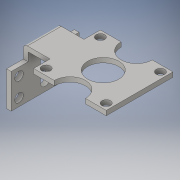
# Autodesk Inventor part: msheehan_motor_mount
Saved by Autodesk Inventor 2016 (Build 200138000, 138)
## iProperties
Created: 2017-08-31
Part Number: msheehan_motor_mount
Material: Generic
Document SubType Name: Modeling
Designer: Student
Density: 1 g/cm^3
Appearance: Default
Author: Student
Autodesk Inventor part; units mm, degrees
ref_plane "YZ Plane" through (0, 0, 0) normal (1, 0, 0) x (0, 1, 0)
ref_plane "XZ Plane" through (0, 0, 0) normal (0, 1, 0) x (-1, 0, 0)
ref_plane "XY Plane" through (0, 0, 0) normal (0, 0, 1) x (1, 0, 0)
sketch "Sketch1" plane through (0, 0, 0) normal (1, 0, 0) x (0, 1, 0)
  line L0 (0, 0) -> (11.176, 0)
  line L1 (11.176, -22.098) -> (0, -22.098)
  line L2 (0, -22.098) -> (0, 0)
  line L3 (11.176, 0) -> (11.176, -5.5245)
  line L4 (11.176, -22.098) -> (11.176, -16.5735)
  line L5 (11.176, -5.5245) -> (15.494, -5.5245)
  line L6 (15.494, -5.5245) -> (15.494, -16.5735)
  line L7 (15.494, -16.5735) -> (11.176, -16.5735)
  line L8 (11.176, 0) -> (11.176, -5.5245)
  line L9 (11.176, -16.5735) -> (11.176, -22.098)
  dimension "d0" = 11.176
  dimension "d1" = 22.098
  dimension "d2" = 5.5245
  dimension "d3" = 5.5245
  dimension "d4" = 4.318
  constraints: 20 end point, 5 perpendicular, 3 parallel, 1 horizontal
  measures "d0" distance of L1.start L1.end
  measures "d1" distance of L0.end L1.start
  measures "d2" distance of L0.end L3.end
  measures "d3" distance of L1.start L4.end
  measures "d4" distance of L3.end L5.end
extrude "Extrusion1" add sketch "Sketch1" along normal blind 1.524
sketch "Sketch2" plane through (1.524, 0, 0) normal (1, 0, 0) x (0, 0, -1)
  line L0 (16.5735, 15.494) -> (5.5245, 15.494) projected
  line L1 (5.5245, 13.97) -> (16.5735, 13.97)
  line L2 (16.5735, 11.176) -> (16.5735, 15.494) projected
  line L3 (16.5735, 13.97) -> (21.9075, 13.97)
  line L4 (21.9075, 13.97) -> (21.9075, 15.494)
  line L5 (21.9075, 15.494) -> (16.5735, 15.494)
  line L6 (5.5245, 15.494) -> (0.1905, 15.494)
  line L7 (0.1905, 15.494) -> (0.1905, 13.97)
  line L8 (0.1905, 13.97) -> (5.5245, 13.97)
  point P0 (0, 0)
  constraints: 14 end point, 4 perpendicular, 2 horizontal
extrude "Extrusion2" add sketch "Sketch2" along normal blind 30.734
fillet "Fillet1" radius 1.27 1 edges at (0, 15.494, -11.049)
fillet "Fillet2" radius 0.254 1 edges at (1.524, 13.97, -11.049)
sketch "Sketch3" plane through (1.524, 0, 0) normal (1, 0, 0) x (0, 0, -1)
  line L0 (22.098, 0) -> (22.098, 11.176) projected
  line L1 (0, 0) -> (22.098, 0) projected
  circle A0 centre (19.558, 2.54) radius 1.397
  line L2 (22.098, 11.176) -> (16.5735, 11.176) projected
  circle A1 centre (19.558, 8.636) radius 1.397
  circle A2 centre (2.54, 2.54) radius 1.397
  circle A3 centre (2.54, 8.636) radius 1.397
  line L3 (11.049, 1.524) -> (11.049, 12.446) construction
  line L4 (12.573, 3.048) -> (12.573, 10.922)
  line L5 (9.525, 10.922) -> (9.525, 3.048)
  arc A4 (9.525, 3.048) -> (12.573, 3.048) centre (11.049, 3.048) ccw
  arc A5 (12.573, 10.922) -> (9.525, 10.922) centre (11.049, 10.922) ccw
  point P0 (11.049, 6.985)
  dimension "d16" = 2.794
  dimension "d19" = 2.794
  dimension "d23" = 10.922
  dimension "d24" = 3.048
  dimension "d50" = 17.018
  constraints: 8 end point, 6 centre point, 6 point on circle, 4 tangent, 2 point on line, 1 midpoint, 1 parallel, 1 vertical
  measures "d16" diameter of A0
  measures "d19" diameter of A1
  measures "d23" distance of L3.start L3.end
  measures "d24" diameter of A5
  measures "d50" distance of A1.centre A3.centre
extrude "Extrusion3" cut sketch "Sketch3" against normal blind 30.734
sketch "Sketch4" plane through (1.524, 15.494, -0.1905) normal (0, 1, 0) x (1, 0, 0)
  line L0 (-1.524, 16.383) -> (0, 16.383) projected
  line L1 (0, 16.383) -> (7.112, 16.383)
  line L2 (-0.254, 5.334) -> (0, 5.334) projected
  line L3 (0, 5.334) -> (7.112, 5.334)
  line L4 (7.112, 16.383) -> (7.112, 21.717)
  line L5 (0, 21.717) -> (30.734, 21.717) projected
  line L6 (7.112, 21.717) -> (0, 21.717)
  line L7 (0, 21.9075) -> (0, 16.383) projected
  line L8 (0, 21.717) -> (0, 16.383)
  line L9 (7.112, 5.334) -> (7.112, 0)
  line L10 (0, 0) -> (30.734, 0) projected
  line L11 (7.112, 0) -> (0, 0)
  line L12 (0, 5.334) -> (0, 16.383) projected
  line L13 (0, 0) -> (0, 5.334)
  point P0 (-1.524, -0.1905)
  dimension "d27" = 7.112
  dimension "d28" = 7.112
  constraints: 16 end point, 2 collinear, 2 horizontal, 2 perpendicular, 2 vertical, 1 point on line
  measures "d27" distance of L0.end L1.end
  measures "d28" distance of L2.end L3.end
extrude "Extrusion4" cut sketch "Sketch4" against normal blind 30.734
sketch "Sketch5" plane through (32.258, 13.97, -21.9075) normal (0, -1, 0) x (1, 0, 0)
  circle A0 centre (-11.811, 10.8585) radius 5.08
  line L0 (-23.622, 21.717) -> (0, 21.717) projected
  circle A1 centre (-11.811, 21.717) radius 5.08
  line L1 (-23.622, 0) -> (0, 0) projected
  circle A2 centre (-11.811, 0) radius 5.08
  point P0 (-32.258, 21.9075)
  dimension "d31" = 10.16
  dimension "d32" = 10.16
  dimension "d33" = 10.16
  constraints: 3 centre point, 2 midpoint
  measures "d31" diameter of A0
  measures "d32" diameter of A1
  measures "d33" diameter of A2
extrude "Extrusion5" cut sketch "Sketch5" against normal blind 30.734
sketch "Sketch6" plane through (32.258, 13.97, -21.9075) normal (0, -1, 0) x (1, 0, 0)
  circle A0 centre (-2.032, 19.685) radius 1.397
  circle A1 centre (-11.811, 10.8585) radius 5.08 projected
  line L0 (0, 21.717) -> (0, 0) projected
  line L1 (0, 0) -> (0, 2.032)
  line L2 (0, 2.032) -> (-2.032, 2.032)
  circle A2 centre (-2.032, 2.032) radius 1.397
  line L3 (-23.622, 21.717) -> (-23.622, 16.383) projected
  line L4 (-23.622, 21.717) -> (-23.622, 19.685)
  line L5 (-23.622, 19.685) -> (-21.59, 19.685)
  circle A3 centre (-21.59, 19.685) radius 1.397
  line L6 (-23.622, 5.334) -> (-23.622, 0) projected
  line L7 (-23.622, 0) -> (-23.622, 2.032)
  line L8 (-23.622, 2.032) -> (-21.59, 2.032)
  circle A4 centre (-21.59, 2.032) radius 1.397
  point P0 (-32.258, 21.9075)
  dimension "d38" = 2.794
  dimension "d39" = 2.032
  dimension "d40" = 2.032
  dimension "d41" = 2.794
  dimension "d42" = 2.032
  dimension "d43" = 2.032
  dimension "d44" = 2.794
  dimension "d45" = 2.032
  dimension "d46" = 2.032
  dimension "d47" = 2.794
  constraints: 12 end point, 4 centre point, 4 coincident, 3 point on line, 2 perpendicular, 1 horizontal
  measures "d38" diameter of A0
  measures "d39" distance of L0.end L1.end
  measures "d40" distance of L1.end L2.end
  measures "d41" diameter of A2
  measures "d42" distance of L3.start L4.end
  measures "d43" distance of L4.end L5.end
  measures "d44" diameter of A3
  measures "d45" distance of L6.end L7.end
  measures "d46" distance of L7.end L8.end
  measures "d47" diameter of A4
extrude "Extrusion6" cut sketch "Sketch6" against normal blind 25.4 contours A0 | A2 | A3 | A4
body "Solid1"
